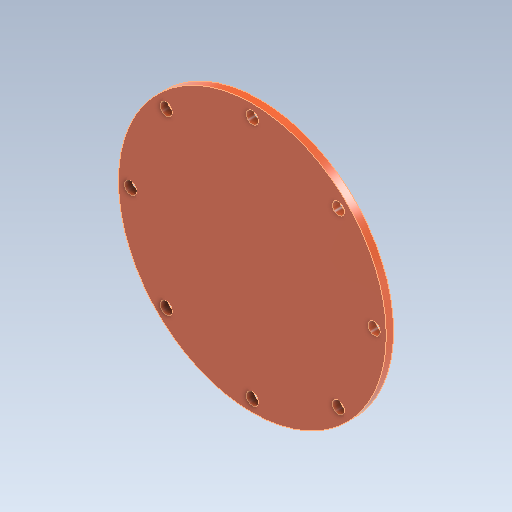
# Autodesk Inventor part: Base3
Saved by Autodesk Inventor 2021 (Build 250183000, 183)
## iProperties
Created: 2021-03-30
Part Number: Base3
Material: Resina fenólica
Document SubType Name: Modeling
Designer: diego
Density: 1.38 g/cm^3
Appearance: Suave - Naranja claro
Author: diego
Autodesk Inventor part; units mm, degrees
ref_plane "YZ Plane" through (0, 0, 0) normal (1, 0, 0) x (0, 1, 0)
ref_plane "XZ Plane" through (0, 0, 0) normal (0, 1, 0) x (-1, 0, 0)
ref_plane "XY Plane" through (0, 0, 0) normal (0, 0, 1) x (1, 0, 0)
sketch "Boceto1" plane through (0, 0, 0) normal (0, 0, 1) x (1, 0, 0)
  circle A0 centre (0, 0) radius 55
  constraints: 1 centre point, 1 coincident
extrude "Extrusión1" add sketch "Boceto1" against normal blind 3
sketch "Boceto2" plane through (0, 0, 0) normal (0, 0, 1) x (1, 0, 0)
  circle A0 centre (0, 50) radius 2.5
  circle A1 centre (-35.3553, 35.3553) radius 2.5
  circle A2 centre (-50, 0) radius 2.5
  circle A3 centre (-35.3553, -35.3553) radius 2.5
  circle A4 centre (0, -50) radius 2.5
  circle A5 centre (35.3553, -35.3553) radius 2.5
  circle A6 centre (50, 0) radius 2.5
  circle A7 centre (35.3553, 35.3553) radius 2.5
  point P0 (0, 0)
  dimension "d7" = 360
  constraints: 8 centre point, 17 other
hole "Agujero1" at (0, 50, 0) at (-35.3553, 35.3553, 0) at (-50, 0, 0) at (-35.3553, -35.3553, 0) at (0, -50, 0) at (35.3553, -35.3553, 0) at (50, 0, 0) at (35.3553, 35.3553, 0) direction (0, 0, -1) diameter 5 end through all
